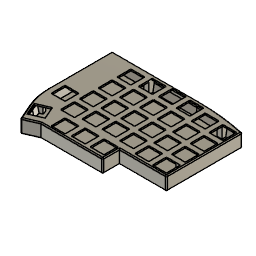
Like Lily58 (Autodesk Fusion 360 design; units mm, degrees)
Autodesk Fusion 360 part; units mm, degrees
(part 1 of 2)
sketch "Plate" plane through (0, 0, 0) normal (0, 0, 1) x (1, 0, 0)
  arc A0 (259.7, -60.0305) -> (260.2, -60.5305) centre (260.2, -60.0305) ccw
  arc A1 (235.6, -61.318) -> (235.1, -60.818) centre (235.1, -61.318) ccw
  line L0 (221.6, -61.318) -> (221.6, -74.318)
  line L1 (222.1, -60.818) -> (235.1, -60.818)
  arc A2 (197, -74.818) -> (197.5, -74.318) centre (197, -74.318) ccw
  line L2 (203.05, -73.675) -> (216.05, -73.675)
  line L3 (159.4, -54.46) -> (159.4, -67.46)
  line L4 (184, -60.818) -> (197, -60.818)
  arc A3 (145.9, -53.96) -> (145.4, -54.46) centre (145.9, -54.46) ccw
  line L5 (184, -74.818) -> (197, -74.818)
  arc A4 (184, -60.818) -> (183.5, -61.318) centre (184, -61.318) ccw
  arc A5 (273.2, -60.5305) -> (273.7, -60.0305) centre (273.2, -60.0305) ccw
  line L6 (235.6, -61.318) -> (235.6, -74.318)
  line L7 (183.5, -61.318) -> (183.5, -74.318)
  arc A6 (183.5, -74.318) -> (184, -74.818) centre (184, -74.318) ccw
  arc A7 (197.5, -61.318) -> (197, -60.818) centre (197, -61.318) ccw
  arc A8 (222.1, -60.818) -> (221.6, -61.318) centre (222.1, -61.318) ccw
  line L8 (273.7, -47.0305) -> (273.7, -60.0305)
  arc A9 (216.55, -60.175) -> (216.05, -59.675) centre (216.05, -60.175) ccw
  line L9 (222.1, -74.818) -> (235.1, -74.818)
  line L10 (197.5, -61.318) -> (197.5, -74.318)
  arc A10 (202.55, -73.175) -> (203.05, -73.675) centre (203.05, -73.175) ccw
  line L11 (259.7, -47.0305) -> (259.7, -60.0305)
  line L12 (260.2, -46.5305) -> (273.2, -46.5305)
  arc A11 (260.2, -46.5305) -> (259.7, -47.0305) centre (260.2, -47.0305) ccw
  line L13 (216.55, -60.175) -> (216.55, -73.175)
  arc A12 (203.05, -59.675) -> (202.55, -60.175) centre (203.05, -60.175) ccw
  line L14 (203.05, -16.525) -> (216.05, -16.525)
  line L15 (260.2, -60.5305) -> (273.2, -60.5305)
  arc A13 (216.05, -16.525) -> (216.55, -16.025) centre (216.05, -16.025) ccw
  line L16 (183.5, -4.168) -> (183.5, -17.168)
  line L17 (197.5, -4.168) -> (197.5, -17.168)
  arc A14 (197.5, -4.168) -> (197, -3.668) centre (197, -4.168) ccw
  arc A15 (197, -17.668) -> (197.5, -17.168) centre (197, -17.168) ccw
  line L18 (216.55, -3.025) -> (216.55, -16.025)
  arc A16 (273.7, -47.0305) -> (273.2, -46.5305) centre (273.2, -47.0305) ccw
  arc A17 (145.4, -67.46) -> (145.9, -67.96) centre (145.9, -67.46) ccw
  arc A18 (159.4, -54.46) -> (158.9, -53.96) centre (158.9, -54.46) ccw
  arc A19 (203.05, -2.525) -> (202.55, -3.025) centre (203.05, -3.025) ccw
  arc A20 (216.55, -3.025) -> (216.05, -2.525) centre (216.05, -3.025) ccw
  arc A21 (158.9, -67.96) -> (159.4, -67.46) centre (158.9, -67.46) ccw
  line L19 (145.9, -67.96) -> (158.9, -67.96)
  line L20 (145.4, -54.46) -> (145.4, -67.46)
  line L21 (145.9, -53.96) -> (158.9, -53.96)
  line L22 (222.1, -3.668) -> (235.1, -3.668)
  line L23 (203.05, -59.675) -> (216.05, -59.675)
  arc A22 (216.05, -73.675) -> (216.55, -73.175) centre (216.05, -73.175) ccw
  line L24 (203.05, -2.525) -> (216.05, -2.525)
  line L25 (184, -3.668) -> (197, -3.668)
  line L26 (202.55, -3.025) -> (202.55, -16.025)
  line L27 (202.55, -60.175) -> (202.55, -73.175)
  line L28 (260.2, -22.4305) -> (273.2, -22.4305)
  line L29 (235.6, -4.168) -> (235.6, -17.168)
  line L30 (164.95, -6.335) -> (177.95, -6.335)
  arc A23 (177.95, -20.335) -> (178.45, -19.835) centre (177.95, -19.835) ccw
  arc A24 (241.15, -7.2875) -> (240.65, -7.7875) centre (241.15, -7.7875) ccw
  line L31 (260.2, -8.4305) -> (273.2, -8.4305)
  line L32 (241.15, -7.2875) -> (254.15, -7.2875)
  line L33 (164.45, -6.835) -> (164.45, -19.835)
  arc A25 (259.7, -21.9305) -> (260.2, -22.4305) centre (260.2, -21.9305) ccw
  arc A26 (222.1, -3.668) -> (221.6, -4.168) centre (222.1, -4.168) ccw
  line L34 (259.7, -8.9305) -> (259.7, -21.9305)
  line L35 (178.45, -6.835) -> (178.45, -19.835)
  line L36 (273.7, -8.9305) -> (273.7, -21.9305)
  arc A27 (254.15, -21.2875) -> (254.65, -20.7875) centre (254.15, -20.7875) ccw
  arc A28 (240.65, -20.7875) -> (241.15, -21.2875) centre (241.15, -20.7875) ccw
  line L37 (221.6, -4.168) -> (221.6, -17.168)
  line L38 (164.95, -20.335) -> (177.95, -20.335)
  arc A29 (254.65, -7.7875) -> (254.15, -7.2875) centre (254.15, -7.7875) ccw
  arc A30 (184, -3.668) -> (183.5, -4.168) centre (184, -4.168) ccw
  line L39 (241.15, -21.2875) -> (254.15, -21.2875)
  arc A31 (164.45, -19.835) -> (164.95, -20.335) centre (164.95, -19.835) ccw
  line L40 (222.1, -17.668) -> (235.1, -17.668)
  arc A32 (178.45, -6.835) -> (177.95, -6.335) centre (177.95, -6.835) ccw
  arc A33 (273.2, -22.4305) -> (273.7, -21.9305) centre (273.2, -21.9305) ccw
  arc A34 (221.6, -17.168) -> (222.1, -17.668) centre (222.1, -17.168) ccw
  arc A35 (235.1, -17.668) -> (235.6, -17.168) centre (235.1, -17.168) ccw
  arc A36 (202.55, -16.025) -> (203.05, -16.525) centre (203.05, -16.025) ccw
  arc A37 (273.7, -8.9305) -> (273.2, -8.4305) centre (273.2, -8.9305) ccw
  arc A38 (164.95, -6.335) -> (164.45, -6.835) centre (164.95, -6.835) ccw
  line L41 (184, -17.668) -> (197, -17.668)
  arc A39 (235.6, -4.168) -> (235.1, -3.668) centre (235.1, -4.168) ccw
  line L42 (240.65, -7.7875) -> (240.65, -20.7875)
  line L43 (254.65, -7.7875) -> (254.65, -20.7875)
  arc A40 (183.5, -17.168) -> (184, -17.668) centre (184, -17.168) ccw
  line L44 (164.45, -25.885) -> (164.45, -38.885)
  arc A41 (164.95, -25.385) -> (164.45, -25.885) centre (164.95, -25.885) ccw
  arc A42 (197, -36.718) -> (197.5, -36.218) centre (197, -36.218) ccw
  arc A43 (178.45, -25.885) -> (177.95, -25.385) centre (177.95, -25.885) ccw
  arc A44 (222.1, -22.718) -> (221.6, -23.218) centre (222.1, -23.218) ccw
  arc A45 (177.95, -39.385) -> (178.45, -38.885) centre (177.95, -38.885) ccw
  arc A46 (260.2, -8.4305) -> (259.7, -8.9305) centre (260.2, -8.9305) ccw
  line L45 (216.55, -22.075) -> (216.55, -35.075)
  line L46 (183.5, -23.218) -> (183.5, -36.218)
  line L47 (203.05, -21.575) -> (216.05, -21.575)
  line L48 (222.1, -36.718) -> (235.1, -36.718)
  arc A47 (197.5, -23.218) -> (197, -22.718) centre (197, -23.218) ccw
  line L49 (164.95, -39.385) -> (177.95, -39.385)
  arc A48 (216.05, -35.575) -> (216.55, -35.075) centre (216.05, -35.075) ccw
  line L50 (178.45, -25.885) -> (178.45, -38.885)
  arc A49 (202.55, -35.075) -> (203.05, -35.575) centre (203.05, -35.075) ccw
  arc A50 (183.5, -36.218) -> (184, -36.718) centre (184, -36.218) ccw
  line L51 (184, -36.718) -> (197, -36.718)
  arc A51 (235.6, -23.218) -> (235.1, -22.718) centre (235.1, -23.218) ccw
  line L52 (222.1, -22.718) -> (235.1, -22.718)
  arc A52 (203.05, -21.575) -> (202.55, -22.075) centre (203.05, -22.075) ccw
  arc A53 (235.1, -36.718) -> (235.6, -36.218) centre (235.1, -36.218) ccw
  line L53 (164.95, -25.385) -> (177.95, -25.385)
  arc A54 (184, -22.718) -> (183.5, -23.218) centre (184, -23.218) ccw
  line L54 (235.6, -23.218) -> (235.6, -36.218)
  line L55 (203.05, -35.575) -> (216.05, -35.575)
  arc A55 (216.55, -22.075) -> (216.05, -21.575) centre (216.05, -22.075) ccw
  line L56 (197.5, -23.218) -> (197.5, -36.218)
  line L57 (184, -22.718) -> (197, -22.718)
  arc A56 (164.45, -38.885) -> (164.95, -39.385) centre (164.95, -38.885) ccw
  line L58 (221.6, -23.218) -> (221.6, -36.218)
  line L59 (216.55, -41.125) -> (216.55, -54.125)
  arc A57 (216.05, -54.625) -> (216.55, -54.125) centre (216.05, -54.125) ccw
  arc A58 (259.7, -40.9805) -> (260.2, -41.4805) centre (260.2, -40.9805) ccw
  line L60 (241.15, -40.3375) -> (254.15, -40.3375)
  line L61 (203.05, -54.625) -> (216.05, -54.625)
  line L62 (202.55, -22.075) -> (202.55, -35.075)
  arc A59 (273.7, -27.9805) -> (273.2, -27.4805) centre (273.2, -27.9805) ccw
  line L63 (184, -55.768) -> (197, -55.768)
  line L64 (260.2, -41.4805) -> (273.2, -41.4805)
  line L65 (259.7, -27.9805) -> (259.7, -40.9805)
  arc A60 (202.55, -54.125) -> (203.05, -54.625) centre (203.05, -54.125) ccw
  arc A61 (203.05, -40.625) -> (202.55, -41.125) centre (203.05, -41.125) ccw
  arc A62 (254.15, -40.3375) -> (254.65, -39.8375) centre (254.15, -39.8375) ccw
  line L66 (240.65, -26.8375) -> (240.65, -39.8375)
  arc A63 (221.6, -36.218) -> (222.1, -36.718) centre (222.1, -36.218) ccw
  arc A64 (240.65, -39.8375) -> (241.15, -40.3375) centre (241.15, -39.8375) ccw
  line L67 (203.05, -40.625) -> (216.05, -40.625)
  arc A65 (273.2, -41.4805) -> (273.7, -40.9805) centre (273.2, -40.9805) ccw
  line L68 (241.15, -26.3375) -> (254.15, -26.3375)
  arc A66 (254.65, -26.8375) -> (254.15, -26.3375) centre (254.15, -26.8375) ccw
  line L69 (184, -41.768) -> (197, -41.768)
  line L70 (183.5, -42.268) -> (183.5, -55.268)
  line L71 (197.5, -42.268) -> (197.5, -55.268)
  arc A67 (216.55, -41.125) -> (216.05, -40.625) centre (216.05, -41.125) ccw
  arc A68 (184, -41.768) -> (183.5, -42.268) centre (184, -42.268) ccw
  line L72 (273.7, -27.9805) -> (273.7, -40.9805)
  arc A69 (260.2, -27.4805) -> (259.7, -27.9805) centre (260.2, -27.9805) ccw
  arc A70 (241.15, -26.3375) -> (240.65, -26.8375) centre (241.15, -26.8375) ccw
  line L73 (202.55, -41.125) -> (202.55, -54.125)
  arc A71 (177.95, -58.435) -> (178.45, -57.935) centre (177.95, -57.935) ccw
  arc A72 (221.6, -55.268) -> (222.1, -55.768) centre (222.1, -55.268) ccw
  line L74 (164.45, -44.935) -> (164.45, -57.935)
  line L75 (241.15, -45.3875) -> (254.15, -45.3875)
  arc A73 (235.1, -55.768) -> (235.6, -55.268) centre (235.1, -55.268) ccw
  line L76 (241.15, -59.3875) -> (254.15, -59.3875)
  line L77 (254.65, -45.8875) -> (254.65, -58.8875)
  line L78 (164.95, -44.435) -> (177.95, -44.435)
  arc A74 (240.65, -58.8875) -> (241.15, -59.3875) centre (241.15, -58.8875) ccw
  line L79 (178.45, -44.935) -> (178.45, -57.935)
  line L80 (222.1, -41.768) -> (235.1, -41.768)
  line L81 (254.65, -26.8375) -> (254.65, -39.8375)
  line L82 (240.65, -45.8875) -> (240.65, -58.8875)
  arc A75 (178.45, -44.935) -> (177.95, -44.435) centre (177.95, -44.935) ccw
  line L83 (222.1, -55.768) -> (235.1, -55.768)
  line L84 (164.95, -58.435) -> (177.95, -58.435)
  arc A76 (254.65, -45.8875) -> (254.15, -45.3875) centre (254.15, -45.8875) ccw
  line L85 (235.6, -42.268) -> (235.6, -55.268)
  arc A77 (183.5, -55.268) -> (184, -55.768) centre (184, -55.268) ccw
  arc A78 (241.15, -45.3875) -> (240.65, -45.8875) centre (241.15, -45.8875) ccw
  arc A79 (235.6, -42.268) -> (235.1, -41.768) centre (235.1, -42.268) ccw
  arc A80 (222.1, -41.768) -> (221.6, -42.268) centre (222.1, -42.268) ccw
  arc A81 (164.45, -57.935) -> (164.95, -58.435) centre (164.95, -57.935) ccw
  line L86 (221.6, -42.268) -> (221.6, -55.268)
  line L87 (260.2, -27.4805) -> (273.2, -27.4805)
  arc A82 (254.15, -59.3875) -> (254.65, -58.8875) centre (254.15, -58.8875) ccw
  arc A83 (177.95, -77.485) -> (178.45, -76.985) centre (177.95, -76.985) ccw
  arc A84 (197.5, -42.268) -> (197, -41.768) centre (197, -42.268) ccw
  line L88 (241.15, -64.4375) -> (254.15, -64.4375)
  arc A85 (273.7, -66.0805) -> (273.2, -65.5805) centre (273.2, -66.0805) ccw
  line L89 (164.95, -63.485) -> (177.95, -63.485)
  arc A86 (197, -55.768) -> (197.5, -55.268) centre (197, -55.268) ccw
  arc A87 (178.45, -63.985) -> (177.95, -63.485) centre (177.95, -63.985) ccw
  line L90 (260.2, -65.5805) -> (273.2, -65.5805)
  arc A88 (164.95, -44.435) -> (164.45, -44.935) centre (164.95, -44.935) ccw
  arc A89 (260.2, -65.5805) -> (259.7, -66.0805) centre (260.2, -66.0805) ccw
  line L91 (241.15, -78.4375) -> (254.15, -78.4375)
  arc A90 (259.7, -79.0805) -> (260.2, -79.5805) centre (260.2, -79.0805) ccw
  line L92 (254.65, -64.9375) -> (254.65, -77.9375)
  line L93 (164.45, -63.985) -> (164.45, -76.985)
  arc A91 (221.6, -74.318) -> (222.1, -74.818) centre (222.1, -74.318) ccw
  arc A92 (235.1, -74.818) -> (235.6, -74.318) centre (235.1, -74.318) ccw
  line L94 (164.95, -77.485) -> (177.95, -77.485)
  line L95 (178.45, -63.985) -> (178.45, -76.985)
  line L96 (259.7, -66.0805) -> (259.7, -79.0805)
  arc A93 (241.15, -64.4375) -> (240.65, -64.9375) centre (241.15, -64.9375) ccw
  line L97 (273.7, -66.0805) -> (273.7, -79.0805)
  arc A94 (164.95, -63.485) -> (164.45, -63.985) centre (164.95, -63.985) ccw
  arc A95 (254.65, -64.9375) -> (254.15, -64.4375) centre (254.15, -64.9375) ccw
  arc A96 (273.2, -79.5805) -> (273.7, -79.0805) centre (273.2, -79.0805) ccw
  arc A97 (254.15, -78.4375) -> (254.65, -77.9375) centre (254.15, -77.9375) ccw
  line L98 (240.65, -64.9375) -> (240.65, -77.9375)
  arc A98 (164.45, -76.985) -> (164.95, -77.485) centre (164.95, -76.985) ccw
  line L99 (260.2, -79.5805) -> (273.2, -79.5805)
  arc A99 (240.65, -77.9375) -> (241.15, -78.4375) centre (241.15, -77.9375) ccw
  line L100 (193.525, -81.2015) -> (206.525, -81.2015)
  line L101 (187.975, -83.035) -> (187.975, -96.035)
  arc A100 (193.025, -94.7015) -> (193.525, -95.2015) centre (193.525, -94.7015) ccw
  arc A101 (187.975, -83.035) -> (187.475, -82.535) centre (187.475, -83.035) ccw
  arc A102 (206.525, -95.2015) -> (207.025, -94.7015) centre (206.525, -94.7015) ccw
  line L102 (174.475, -82.535) -> (187.475, -82.535)
  arc A103 (225.575, -95.2015) -> (226.075, -94.7015) centre (225.575, -94.7015) ccw
  line L103 (212.575, -81.2015) -> (225.575, -81.2015)
  arc A104 (212.075, -94.7015) -> (212.575, -95.2015) centre (212.575, -94.7015) ccw
  line L104 (193.025, -81.7015) -> (193.025, -94.7015)
  arc A105 (174.475, -82.535) -> (173.975, -83.035) centre (174.475, -83.035) ccw
  line L105 (173.975, -83.035) -> (173.975, -96.035)
  arc A106 (207.025, -81.7015) -> (206.525, -81.2015) centre (206.525, -81.7015) ccw
  line L106 (207.025, -81.7015) -> (207.025, -94.7015)
  arc A107 (226.075, -81.7015) -> (225.575, -81.2015) centre (225.575, -81.7015) ccw
  line L107 (212.075, -81.7015) -> (212.075, -94.7015)
  line L108 (212.575, -95.2015) -> (225.575, -95.2015)
  arc A108 (187.475, -96.535) -> (187.975, -96.035) centre (187.475, -96.035) ccw
  arc A109 (173.975, -96.035) -> (174.475, -96.535) centre (174.475, -96.035) ccw
  arc A110 (193.525, -81.2015) -> (193.025, -81.7015) centre (193.525, -81.7015) ccw
  line L109 (174.475, -96.535) -> (187.475, -96.535)
  line L110 (226.075, -81.7015) -> (226.075, -94.7015)
  arc A111 (212.575, -81.2015) -> (212.075, -81.7015) centre (212.575, -81.7015) ccw
  line L111 (193.525, -95.2015) -> (206.525, -95.2015)
  line L112 (226.8375, -0.025) -> (139.1942, -0.025)
  line L113 (276.2, -82.0805) -> (276.2, -5.454)
  arc A112 (276.2, -5.454) -> (226.8375, -0.025) centre (226.8375, -227.1492) ccw
  line L114 (276.2, -82.0805) -> (228.575, -82.0805)
  line L115 (165.9817, -99.035) -> (228.575, -99.035)
  line L116 (228.575, -99.035) -> (228.575, -82.0805)
  line L117 (145.666, -85.4803) -> (158.518, -79.9282)
  line L118 (158.518, -79.9282) -> (164.0701, -92.7802)
  line L119 (164.0701, -92.7802) -> (151.218, -98.3323)
  line L120 (151.218, -98.3323) -> (145.666, -85.4803)
  line L121 (139.1942, -0.025) -> (139.1942, -64.9159)
  line L122 (165.9817, -99.035) -> (151.5008, -105.2907)
  line L123 (151.5008, -105.2907) -> (143.9083, -87.7156)
  arc A113 (139.1942, -64.9159) -> (143.9083, -87.7156) centre (196.6857, -64.9159) ccw
  dimension "d8" = 2.5
  dimension "d9" = 2.5
  dimension "d11" = 2.5
  dimension "d12" = 2.5
  dimension "d13" = 2.5
  dimension "d24" = 2.5
  dimension "d29" = 6.5
  constraint tangent L112 A112
  constraint parallel L24 L112
  constraint perpendicular L113 L114
  constraint horizontal L115
  constraint perpendicular L114 L116
  constraint perpendicular L112 L121
  constraint tangent L123 A113
  constraint tangent L121 A113
  constraint parallel L120 L123
  constraint parallel L119 L122
  measures "d8" distance of L24 L112
  measures "d9" distance of L72 L113
  measures "d11" distance of L109 L115
  measures "d12" distance of L110 L116
  measures "d13" distance of L99 L114
  measures "d24" distance of L120 L123
  measures "d29" distance of L119 L122
extrude "Extrude1" add sketch "Plate" against normal blind 3.5 thin wall 1.7 inside contours A0 A5 L8 L11 L12 A11 L15 A16 | A1 L0 L1 L6 A8 L9 A91 A92 | A2 L4 L5 A4 L7 A6 A7 L10 | L2 A9 A10 L13 A12 L23 A22 L27 | L3 A3 A17 A18 A21 L19 L20 L21 | L14 A13 L18 A19 A20 L24 L26 A36 | L16 L17 A14 A15 L25 A30 L41 A40 | L22 L29 A26 L37 L40 A34 A35 A39 | L28 L31 A25 L34 L36 A33 A37 A46 | L30 A23 L33 L35 L38 A31 A32 A38 | A24 L32 A27 A28 A29 L39 L42 L43 | L44 A41 A43 A45 L49 L50 L53 A56 | A42 L46 A47 A50 L51 A54 L56 L57 | A44 L48 A51 L52 A53 L54 L58 A63 | L45 L47 A48 A49 A52 L55 A55 L62 | L59 A57 L61 A60 A61 L67 A67 L73 | A58 A59 L64 L65 A65 L72 A69 L87 | L60 A62 L66 A64 L68 A66 A70 L81 | L63 L69 L70 L71 A68 A77 A84 A86 | A71 L74 L78 L79 A75 L84 A81 A88 | A72 A73 L80 L83 L85 A79 A80 L86 | L75 L76 L77 A74 L82 A76 A78 A82 | A83 L89 A87 L93 L94 L95 A94 A98 | L88 L91 L92 A93 A95 A97 L98 A99 | A85 L90 A89 A90 L96 L97 A96 L99 | L100 A100 A102 L104 A106 L106 A110 L111 | L101 A101 L102 A105 L105 A108 A109 L109 | A103 L103 A104 A107 L107 L108 L110 A111 | L112 L113 A112 L114 L115 L116 L121 L122 L123 A113 | L117 L118 L119 L120 makes body 1
extrude "Extrude2" add sketch "Plate" along normal blind 1.5 bodies 1
extrude "Extrude3" add 1 faces at (168.9753, -0.5917, -3.5) along direction (0, 0, -1) blind 7.5 draft 10 on bodies 1 bodies 1
sketch "Sketch5" plane through (0, 0, 1.5) normal (0, 0, 1) x (-1, 0, 0)
  line L0 (-164.0701, 92.7802) -> (-151.218, 98.3323)
  line L1 (-151.218, 98.3323) -> (-145.666, 85.4803)
  line L2 (-145.666, 85.4803) -> (-158.518, 79.9282)
  line L3 (-158.518, 79.9282) -> (-164.0701, 92.7802)
  arc A0 (-260.2, 65.5805) -> (-259.7, 66.0805) centre (-260.2, 66.0805) ccw
  line L4 (-260.2, 65.5805) -> (-273.2, 65.5805)
  arc A1 (-273.7, 66.0805) -> (-273.2, 65.5805) centre (-273.2, 66.0805) ccw
  line L5 (-273.7, 66.0805) -> (-273.7, 79.0805)
  arc A2 (-273.2, 79.5805) -> (-273.7, 79.0805) centre (-273.2, 79.0805) ccw
  line L6 (-273.2, 79.5805) -> (-260.2, 79.5805)
  arc A3 (-259.7, 79.0805) -> (-260.2, 79.5805) centre (-260.2, 79.0805) ccw
  line L7 (-259.7, 79.0805) -> (-259.7, 66.0805)
  arc A4 (-174.475, 82.535) -> (-173.975, 83.035) centre (-174.475, 83.035) ccw
  line L8 (-174.475, 82.535) -> (-187.475, 82.535)
  arc A5 (-187.975, 83.035) -> (-187.475, 82.535) centre (-187.475, 83.035) ccw
  line L9 (-187.975, 83.035) -> (-187.975, 96.035)
  arc A6 (-187.475, 96.535) -> (-187.975, 96.035) centre (-187.475, 96.035) ccw
  line L10 (-187.475, 96.535) -> (-174.475, 96.535)
  arc A7 (-173.975, 96.035) -> (-174.475, 96.535) centre (-174.475, 96.035) ccw
  line L11 (-173.975, 96.035) -> (-173.975, 83.035)
  arc A8 (-203.05, 59.675) -> (-202.55, 60.175) centre (-203.05, 60.175) ccw
  line L12 (-203.05, 59.675) -> (-216.05, 59.675)
  arc A9 (-216.55, 60.175) -> (-216.05, 59.675) centre (-216.05, 60.175) ccw
  line L13 (-216.55, 60.175) -> (-216.55, 73.175)
  arc A10 (-216.05, 73.675) -> (-216.55, 73.175) centre (-216.05, 73.175) ccw
  line L14 (-216.05, 73.675) -> (-203.05, 73.675)
  arc A11 (-202.55, 73.175) -> (-203.05, 73.675) centre (-203.05, 73.175) ccw
  line L15 (-202.55, 73.175) -> (-202.55, 60.175)
  arc A12 (-260.2, 46.5305) -> (-259.7, 47.0305) centre (-260.2, 47.0305) ccw
  line L16 (-260.2, 46.5305) -> (-273.2, 46.5305)
  arc A13 (-273.7, 47.0305) -> (-273.2, 46.5305) centre (-273.2, 47.0305) ccw
  line L17 (-273.7, 47.0305) -> (-273.7, 60.0305)
  arc A14 (-273.2, 60.5305) -> (-273.7, 60.0305) centre (-273.2, 60.0305) ccw
  line L18 (-273.2, 60.5305) -> (-260.2, 60.5305)
  arc A15 (-259.7, 60.0305) -> (-260.2, 60.5305) centre (-260.2, 60.0305) ccw
  line L19 (-259.7, 60.0305) -> (-259.7, 47.0305)
  arc A16 (-241.15, 64.4375) -> (-240.65, 64.9375) centre (-241.15, 64.9375) ccw
  line L20 (-241.15, 64.4375) -> (-254.15, 64.4375)
  arc A17 (-254.65, 64.9375) -> (-254.15, 64.4375) centre (-254.15, 64.9375) ccw
  line L21 (-254.65, 64.9375) -> (-254.65, 77.9375)
  arc A18 (-254.15, 78.4375) -> (-254.65, 77.9375) centre (-254.15, 77.9375) ccw
  line L22 (-254.15, 78.4375) -> (-241.15, 78.4375)
  arc A19 (-240.65, 77.9375) -> (-241.15, 78.4375) centre (-241.15, 77.9375) ccw
  line L23 (-240.65, 77.9375) -> (-240.65, 64.9375)
  arc A20 (-164.95, 63.485) -> (-164.45, 63.985) centre (-164.95, 63.985) ccw
  line L24 (-164.95, 63.485) -> (-177.95, 63.485)
  arc A21 (-178.45, 63.985) -> (-177.95, 63.485) centre (-177.95, 63.985) ccw
  line L25 (-178.45, 63.985) -> (-178.45, 76.985)
  arc A22 (-177.95, 77.485) -> (-178.45, 76.985) centre (-177.95, 76.985) ccw
  line L26 (-177.95, 77.485) -> (-164.95, 77.485)
  arc A23 (-164.45, 76.985) -> (-164.95, 77.485) centre (-164.95, 76.985) ccw
  line L27 (-164.45, 76.985) -> (-164.45, 63.985)
  arc A24 (-222.1, 60.818) -> (-221.6, 61.318) centre (-222.1, 61.318) ccw
  line L28 (-222.1, 60.818) -> (-235.1, 60.818)
  arc A25 (-235.6, 61.318) -> (-235.1, 60.818) centre (-235.1, 61.318) ccw
  line L29 (-235.6, 61.318) -> (-235.6, 74.318)
  arc A26 (-235.1, 74.818) -> (-235.6, 74.318) centre (-235.1, 74.318) ccw
  line L30 (-235.1, 74.818) -> (-222.1, 74.818)
  arc A27 (-221.6, 74.318) -> (-222.1, 74.818) centre (-222.1, 74.318) ccw
  line L31 (-221.6, 74.318) -> (-221.6, 61.318)
  arc A28 (-226.075, 81.7015) -> (-225.575, 81.2015) centre (-225.575, 81.7015) ccw
  line L32 (-226.075, 81.7015) -> (-226.075, 94.7015)
  arc A29 (-225.575, 95.2015) -> (-226.075, 94.7015) centre (-225.575, 94.7015) ccw
  line L33 (-225.575, 95.2015) -> (-212.575, 95.2015)
  arc A30 (-212.075, 94.7015) -> (-212.575, 95.2015) centre (-212.575, 94.7015) ccw
  line L34 (-212.075, 94.7015) -> (-212.075, 81.7015)
  arc A31 (-212.575, 81.2015) -> (-212.075, 81.7015) centre (-212.575, 81.7015) ccw
  line L35 (-212.575, 81.2015) -> (-225.575, 81.2015)
  arc A32 (-193.525, 81.2015) -> (-193.025, 81.7015) centre (-193.525, 81.7015) ccw
  line L36 (-193.525, 81.2015) -> (-206.525, 81.2015)
  arc A33 (-207.025, 81.7015) -> (-206.525, 81.2015) centre (-206.525, 81.7015) ccw
  line L37 (-207.025, 81.7015) -> (-207.025, 94.7015)
  arc A34 (-206.525, 95.2015) -> (-207.025, 94.7015) centre (-206.525, 94.7015) ccw
  line L38 (-206.525, 95.2015) -> (-193.525, 95.2015)
  arc A35 (-193.025, 94.7015) -> (-193.525, 95.2015) centre (-193.525, 94.7015) ccw
  line L39 (-193.025, 94.7015) -> (-193.025, 81.7015)
  arc A36 (-178.45, 44.935) -> (-177.95, 44.435) centre (-177.95, 44.935) ccw
  line L40 (-178.45, 44.935) -> (-178.45, 57.935)
  arc A37 (-177.95, 58.435) -> (-178.45, 57.935) centre (-177.95, 57.935) ccw
  line L41 (-177.95, 58.435) -> (-164.95, 58.435)
  arc A38 (-164.45, 57.935) -> (-164.95, 58.435) centre (-164.95, 57.935) ccw
  line L42 (-164.45, 57.935) -> (-164.45, 44.935)
  arc A39 (-164.95, 44.435) -> (-164.45, 44.935) centre (-164.95, 44.935) ccw
  line L43 (-164.95, 44.435) -> (-177.95, 44.435)
  arc A40 (-241.15, 45.3875) -> (-240.65, 45.8875) centre (-241.15, 45.8875) ccw
  line L44 (-241.15, 45.3875) -> (-254.15, 45.3875)
  arc A41 (-254.65, 45.8875) -> (-254.15, 45.3875) centre (-254.15, 45.8875) ccw
  line L45 (-254.65, 45.8875) -> (-254.65, 58.8875)
  arc A42 (-254.15, 59.3875) -> (-254.65, 58.8875) centre (-254.15, 58.8875) ccw
  line L46 (-254.15, 59.3875) -> (-241.15, 59.3875)
  arc A43 (-240.65, 58.8875) -> (-241.15, 59.3875) centre (-241.15, 58.8875) ccw
  line L47 (-240.65, 58.8875) -> (-240.65, 45.8875)
  arc A44 (-184, 41.768) -> (-183.5, 42.268) centre (-184, 42.268) ccw
  line L48 (-184, 41.768) -> (-197, 41.768)
  arc A45 (-197.5, 42.268) -> (-197, 41.768) centre (-197, 42.268) ccw
  line L49 (-197.5, 42.268) -> (-197.5, 55.268)
  arc A46 (-197, 55.768) -> (-197.5, 55.268) centre (-197, 55.268) ccw
  line L50 (-197, 55.768) -> (-184, 55.768)
  arc A47 (-183.5, 55.268) -> (-184, 55.768) centre (-184, 55.268) ccw
  line L51 (-183.5, 55.268) -> (-183.5, 42.268)
  line L52 (-259.7, 40.9805) -> (-259.7, 27.9805)
  arc A48 (-260.2, 27.4805) -> (-259.7, 27.9805) centre (-260.2, 27.9805) ccw
  line L53 (-260.2, 27.4805) -> (-273.2, 27.4805)
  arc A49 (-273.7, 27.9805) -> (-273.2, 27.4805) centre (-273.2, 27.9805) ccw
  line L54 (-273.7, 27.9805) -> (-273.7, 40.9805)
  arc A50 (-273.2, 41.4805) -> (-273.7, 40.9805) centre (-273.2, 40.9805) ccw
  line L55 (-273.2, 41.4805) -> (-260.2, 41.4805)
  arc A51 (-259.7, 40.9805) -> (-260.2, 41.4805) centre (-260.2, 40.9805) ccw
  arc A52 (-222.1, 41.768) -> (-221.6, 42.268) centre (-222.1, 42.268) ccw
  line L56 (-222.1, 41.768) -> (-235.1, 41.768)
  arc A53 (-235.6, 42.268) -> (-235.1, 41.768) centre (-235.1, 42.268) ccw
  line L57 (-235.6, 42.268) -> (-235.6, 55.268)
  arc A54 (-235.1, 55.768) -> (-235.6, 55.268) centre (-235.1, 55.268) ccw
  line L58 (-235.1, 55.768) -> (-222.1, 55.768)
  arc A55 (-221.6, 55.268) -> (-222.1, 55.768) centre (-222.1, 55.268) ccw
  line L59 (-221.6, 55.268) -> (-221.6, 42.268)
  arc A56 (-203.05, 40.625) -> (-202.55, 41.125) centre (-203.05, 41.125) ccw
  line L60 (-203.05, 40.625) -> (-216.05, 40.625)
  arc A57 (-216.55, 41.125) -> (-216.05, 40.625) centre (-216.05, 41.125) ccw
  line L61 (-216.55, 41.125) -> (-216.55, 54.125)
  arc A58 (-216.05, 54.625) -> (-216.55, 54.125) centre (-216.05, 54.125) ccw
  line L62 (-216.05, 54.625) -> (-203.05, 54.625)
  arc A59 (-202.55, 54.125) -> (-203.05, 54.625) centre (-203.05, 54.125) ccw
  line L63 (-202.55, 54.125) -> (-202.55, 41.125)
  arc A60 (-222.1, 22.718) -> (-221.6, 23.218) centre (-222.1, 23.218) ccw
  line L64 (-222.1, 22.718) -> (-235.1, 22.718)
  arc A61 (-235.6, 23.218) -> (-235.1, 22.718) centre (-235.1, 23.218) ccw
  line L65 (-235.6, 23.218) -> (-235.6, 36.218)
  arc A62 (-235.1, 36.718) -> (-235.6, 36.218) centre (-235.1, 36.218) ccw
  line L66 (-235.1, 36.718) -> (-222.1, 36.718)
  arc A63 (-221.6, 36.218) -> (-222.1, 36.718) centre (-222.1, 36.218) ccw
  line L67 (-221.6, 36.218) -> (-221.6, 23.218)
  arc A64 (-241.15, 26.3375) -> (-240.65, 26.8375) centre (-241.15, 26.8375) ccw
  line L68 (-241.15, 26.3375) -> (-254.15, 26.3375)
  arc A65 (-254.65, 26.8375) -> (-254.15, 26.3375) centre (-254.15, 26.8375) ccw
  line L69 (-254.65, 26.8375) -> (-254.65, 39.8375)
  arc A66 (-254.15, 40.3375) -> (-254.65, 39.8375) centre (-254.15, 39.8375) ccw
  line L70 (-254.15, 40.3375) -> (-241.15, 40.3375)
  arc A67 (-240.65, 39.8375) -> (-241.15, 40.3375) centre (-241.15, 39.8375) ccw
  line L71 (-240.65, 39.8375) -> (-240.65, 26.8375)
  arc A68 (-203.05, 21.575) -> (-202.55, 22.075) centre (-203.05, 22.075) ccw
  line L72 (-203.05, 21.575) -> (-216.05, 21.575)
  arc A69 (-216.55, 22.075) -> (-216.05, 21.575) centre (-216.05, 22.075) ccw
  line L73 (-216.55, 22.075) -> (-216.55, 35.075)
  arc A70 (-216.05, 35.575) -> (-216.55, 35.075) centre (-216.05, 35.075) ccw
  line L74 (-216.05, 35.575) -> (-203.05, 35.575)
  arc A71 (-202.55, 35.075) -> (-203.05, 35.575) centre (-203.05, 35.075) ccw
  line L75 (-202.55, 35.075) -> (-202.55, 22.075)
  arc A72 (-164.95, 25.385) -> (-164.45, 25.885) centre (-164.95, 25.885) ccw
  line L76 (-164.95, 25.385) -> (-177.95, 25.385)
  arc A73 (-178.45, 25.885) -> (-177.95, 25.385) centre (-177.95, 25.885) ccw
  line L77 (-178.45, 25.885) -> (-178.45, 38.885)
  arc A74 (-177.95, 39.385) -> (-178.45, 38.885) centre (-177.95, 38.885) ccw
  line L78 (-177.95, 39.385) -> (-164.95, 39.385)
  arc A75 (-164.45, 38.885) -> (-164.95, 39.385) centre (-164.95, 38.885) ccw
  line L79 (-164.45, 38.885) -> (-164.45, 25.885)
  line L80 (-183.5, 36.218) -> (-183.5, 23.218)
  arc A76 (-184, 22.718) -> (-183.5, 23.218) centre (-184, 23.218) ccw
  line L81 (-184, 22.718) -> (-197, 22.718)
  arc A77 (-197.5, 23.218) -> (-197, 22.718) centre (-197, 23.218) ccw
  line L82 (-197.5, 23.218) -> (-197.5, 36.218)
  arc A78 (-197, 36.718) -> (-197.5, 36.218) centre (-197, 36.218) ccw
  line L83 (-197, 36.718) -> (-184, 36.718)
  arc A79 (-183.5, 36.218) -> (-184, 36.718) centre (-184, 36.218) ccw
  arc A80 (-184, 60.818) -> (-183.5, 61.318) centre (-184, 61.318) ccw
  line L84 (-184, 60.818) -> (-197, 60.818)
  arc A81 (-197.5, 61.318) -> (-197, 60.818) centre (-197, 61.318) ccw
  line L85 (-197.5, 61.318) -> (-197.5, 74.318)
  arc A82 (-197, 74.818) -> (-197.5, 74.318) centre (-197, 74.318) ccw
  line L86 (-197, 74.818) -> (-184, 74.818)
  arc A83 (-183.5, 74.318) -> (-184, 74.818) centre (-184, 74.318) ccw
  line L87 (-183.5, 74.318) -> (-183.5, 61.318)
  line L88 (-145.4, 67.46) -> (-145.4, 54.46)
  arc A84 (-145.9, 53.96) -> (-145.4, 54.46) centre (-145.9, 54.46) ccw
  line L89 (-145.9, 53.96) -> (-158.9, 53.96)
  arc A85 (-159.4, 54.46) -> (-158.9, 53.96) centre (-158.9, 54.46) ccw
  line L90 (-159.4, 54.46) -> (-159.4, 67.46)
  arc A86 (-158.9, 67.96) -> (-159.4, 67.46) centre (-158.9, 67.46) ccw
  line L91 (-158.9, 67.96) -> (-145.9, 67.96)
  arc A87 (-145.4, 67.46) -> (-145.9, 67.96) centre (-145.9, 67.46) ccw
  arc A88 (-241.15, 7.2875) -> (-240.65, 7.7875) centre (-241.15, 7.7875) ccw
  line L92 (-241.15, 7.2875) -> (-254.15, 7.2875)
  arc A89 (-254.65, 7.7875) -> (-254.15, 7.2875) centre (-254.15, 7.7875) ccw
  line L93 (-254.65, 7.7875) -> (-254.65, 20.7875)
  arc A90 (-254.15, 21.2875) -> (-254.65, 20.7875) centre (-254.15, 20.7875) ccw
  line L94 (-254.15, 21.2875) -> (-241.15, 21.2875)
  arc A91 (-240.65, 20.7875) -> (-241.15, 21.2875) centre (-241.15, 20.7875) ccw
  line L95 (-240.65, 20.7875) -> (-240.65, 7.7875)
  arc A92 (-222.1, 3.668) -> (-221.6, 4.168) centre (-222.1, 4.168) ccw
  line L96 (-222.1, 3.668) -> (-235.1, 3.668)
  arc A93 (-235.6, 4.168) -> (-235.1, 3.668) centre (-235.1, 4.168) ccw
  line L97 (-235.6, 4.168) -> (-235.6, 17.168)
  arc A94 (-235.1, 17.668) -> (-235.6, 17.168) centre (-235.1, 17.168) ccw
  line L98 (-235.1, 17.668) -> (-222.1, 17.668)
  arc A95 (-221.6, 17.168) -> (-222.1, 17.668) centre (-222.1, 17.168) ccw
  line L99 (-221.6, 17.168) -> (-221.6, 4.168)
  arc A96 (-178.45, 6.835) -> (-177.95, 6.335) centre (-177.95, 6.835) ccw
  line L100 (-178.45, 6.835) -> (-178.45, 19.835)
  arc A97 (-177.95, 20.335) -> (-178.45, 19.835) centre (-177.95, 19.835) ccw
  line L101 (-177.95, 20.335) -> (-164.95, 20.335)
  arc A98 (-164.45, 19.835) -> (-164.95, 20.335) centre (-164.95, 19.835) ccw
  line L102 (-164.45, 19.835) -> (-164.45, 6.835)
  arc A99 (-164.95, 6.335) -> (-164.45, 6.835) centre (-164.95, 6.835) ccw
  line L103 (-164.95, 6.335) -> (-177.95, 6.335)
  arc A100 (-203.05, 2.525) -> (-202.55, 3.025) centre (-203.05, 3.025) ccw
  line L104 (-203.05, 2.525) -> (-216.05, 2.525)
  arc A101 (-216.55, 3.025) -> (-216.05, 2.525) centre (-216.05, 3.025) ccw
  line L105 (-216.55, 3.025) -> (-216.55, 16.025)
  arc A102 (-216.05, 16.525) -> (-216.55, 16.025) centre (-216.05, 16.025) ccw
  line L106 (-216.05, 16.525) -> (-203.05, 16.525)
  arc A103 (-202.55, 16.025) -> (-203.05, 16.525) centre (-203.05, 16.025) ccw
  line L107 (-202.55, 16.025) -> (-202.55, 3.025)
  arc A104 (-273.7, 8.9305) -> (-273.2, 8.4305) centre (-273.2, 8.9305) ccw
  line L108 (-273.7, 8.9305) -> (-273.7, 21.9305)
  arc A105 (-273.2, 22.4305) -> (-273.7, 21.9305) centre (-273.2, 21.9305) ccw
  line L109 (-273.2, 22.4305) -> (-260.2, 22.4305)
  arc A106 (-259.7, 21.9305) -> (-260.2, 22.4305) centre (-260.2, 21.9305) ccw
  line L110 (-259.7, 21.9305) -> (-259.7, 8.9305)
  arc A107 (-260.2, 8.4305) -> (-259.7, 8.9305) centre (-260.2, 8.9305) ccw
  line L111 (-260.2, 8.4305) -> (-273.2, 8.4305)
  arc A108 (-184, 3.668) -> (-183.5, 4.168) centre (-184, 4.168) ccw
  line L112 (-184, 3.668) -> (-197, 3.668)
  arc A109 (-197.5, 4.168) -> (-197, 3.668) centre (-197, 4.168) ccw
  line L113 (-197.5, 4.168) -> (-197.5, 17.168)
  arc A110 (-197, 17.668) -> (-197.5, 17.168) centre (-197, 17.168) ccw
  line L114 (-197, 17.668) -> (-184, 17.668)
  arc A111 (-183.5, 17.168) -> (-184, 17.668) centre (-184, 17.168) ccw
  line L115 (-183.5, 17.168) -> (-183.5, 4.168)
  line L116 (-276.2, 82.0805) -> (-276.2, 5.454)
  arc A112 (-276.2, 5.454) -> (-226.8375, 0.025) centre (-226.8375, 227.1492) ccw
  line L117 (-226.8375, 0.025) -> (-139.1942, 0.025)
  line L118 (-139.1942, 0.025) -> (-139.1942, 64.9159)
  arc A113 (-139.1942, 64.9159) -> (-143.9083, 87.7156) centre (-196.6857, 64.9159) ccw
  line L119 (-143.9083, 87.7156) -> (-151.5008, 105.2907)
  line L120 (-151.5008, 105.2907) -> (-165.9817, 99.035)
  line L121 (-165.9817, 99.035) -> (-228.575, 99.035)
  line L122 (-228.575, 99.035) -> (-228.575, 82.0805)
  line L123 (-228.575, 82.0805) -> (-276.2, 82.0805)
  line L124 (-126.932, -12.1644) -> (-288.3358, -12.1644)
  line L125 (-288.3358, -12.1644) -> (-288.3358, 119.2108)
  line L126 (-288.3358, 119.2108) -> (-126.932, 119.2108)
  line L127 (-126.932, 119.2108) -> (-126.932, -12.1644)
  constraint horizontal L124
  constraint vertical L125
  constraint horizontal L126
  constraint vertical L127
extrude "Extrude4" cut sketch "Sketch5" against normal blind 55 contours L124 L125 L126 L127 bodies 1
sketch "Sketch6" plane through (0, 0, 0) normal (0, 0, -1) x (1, 0, 0)
  arc A0 (183.5, 4.168) -> (184, 3.668) centre (184, 4.168) ccw
  line L0 (183.5, 4.168) -> (183.5, 17.168)
  arc A1 (184, 17.668) -> (183.5, 17.168) centre (184, 17.168) ccw
  line L1 (184, 17.668) -> (197, 17.668)
  arc A2 (197.5, 17.168) -> (197, 17.668) centre (197, 17.168) ccw
  line L2 (197.5, 17.168) -> (197.5, 4.168)
  arc A3 (197, 3.668) -> (197.5, 4.168) centre (197, 4.168) ccw
  line L3 (197, 3.668) -> (184, 3.668)
  arc A4 (273.2, 8.4305) -> (273.7, 8.9305) centre (273.2, 8.9305) ccw
  line L4 (273.2, 8.4305) -> (260.2, 8.4305)
  arc A5 (259.7, 8.9305) -> (260.2, 8.4305) centre (260.2, 8.9305) ccw
  line L5 (259.7, 8.9305) -> (259.7, 21.9305)
  arc A6 (260.2, 22.4305) -> (259.7, 21.9305) centre (260.2, 21.9305) ccw
  line L6 (260.2, 22.4305) -> (273.2, 22.4305)
  arc A7 (273.7, 21.9305) -> (273.2, 22.4305) centre (273.2, 21.9305) ccw
  line L7 (273.7, 21.9305) -> (273.7, 8.9305)
  arc A8 (202.55, 3.025) -> (203.05, 2.525) centre (203.05, 3.025) ccw
  line L8 (202.55, 3.025) -> (202.55, 16.025)
  arc A9 (203.05, 16.525) -> (202.55, 16.025) centre (203.05, 16.025) ccw
  line L9 (203.05, 16.525) -> (216.05, 16.525)
  arc A10 (216.55, 16.025) -> (216.05, 16.525) centre (216.05, 16.025) ccw
  line L10 (216.55, 16.025) -> (216.55, 3.025)
  arc A11 (216.05, 2.525) -> (216.55, 3.025) centre (216.05, 3.025) ccw
  line L11 (216.05, 2.525) -> (203.05, 2.525)
  arc A12 (177.95, 6.335) -> (178.45, 6.835) centre (177.95, 6.835) ccw
  line L12 (177.95, 6.335) -> (164.95, 6.335)
  arc A13 (164.45, 6.835) -> (164.95, 6.335) centre (164.95, 6.835) ccw
  line L13 (164.45, 6.835) -> (164.45, 19.835)
  arc A14 (164.95, 20.335) -> (164.45, 19.835) centre (164.95, 19.835) ccw
  line L14 (164.95, 20.335) -> (177.95, 20.335)
  arc A15 (178.45, 19.835) -> (177.95, 20.335) centre (177.95, 19.835) ccw
  line L15 (178.45, 19.835) -> (178.45, 6.835)
  arc A16 (221.6, 4.168) -> (222.1, 3.668) centre (222.1, 4.168) ccw
  line L16 (221.6, 4.168) -> (221.6, 17.168)
  arc A17 (222.1, 17.668) -> (221.6, 17.168) centre (222.1, 17.168) ccw
  line L17 (222.1, 17.668) -> (235.1, 17.668)
  arc A18 (235.6, 17.168) -> (235.1, 17.668) centre (235.1, 17.168) ccw
  line L18 (235.6, 17.168) -> (235.6, 4.168)
  arc A19 (235.1, 3.668) -> (235.6, 4.168) centre (235.1, 4.168) ccw
  line L19 (235.1, 3.668) -> (222.1, 3.668)
  arc A20 (240.65, 7.7875) -> (241.15, 7.2875) centre (241.15, 7.7875) ccw
  line L20 (240.65, 7.7875) -> (240.65, 20.7875)
  arc A21 (241.15, 21.2875) -> (240.65, 20.7875) centre (241.15, 20.7875) ccw
  line L21 (241.15, 21.2875) -> (254.15, 21.2875)
  arc A22 (254.65, 20.7875) -> (254.15, 21.2875) centre (254.15, 20.7875) ccw
  line L22 (254.65, 20.7875) -> (254.65, 7.7875)
  arc A23 (254.15, 7.2875) -> (254.65, 7.7875) centre (254.15, 7.7875) ccw
  line L23 (254.15, 7.2875) -> (241.15, 7.2875)
  line L24 (145.4, 54.46) -> (145.4, 67.46)
  arc A24 (145.9, 67.96) -> (145.4, 67.46) centre (145.9, 67.46) ccw
  line L25 (145.9, 67.96) -> (158.9, 67.96)
  arc A25 (159.4, 67.46) -> (158.9, 67.96) centre (158.9, 67.46) ccw
  line L26 (159.4, 67.46) -> (159.4, 54.46)
  arc A26 (158.9, 53.96) -> (159.4, 54.46) centre (158.9, 54.46) ccw
  line L27 (158.9, 53.96) -> (145.9, 53.96)
  arc A27 (145.4, 54.46) -> (145.9, 53.96) centre (145.9, 54.46) ccw
  arc A28 (183.5, 61.318) -> (184, 60.818) centre (184, 61.318) ccw
  line L28 (183.5, 61.318) -> (183.5, 74.318)
  arc A29 (184, 74.818) -> (183.5, 74.318) centre (184, 74.318) ccw
  line L29 (184, 74.818) -> (197, 74.818)
  arc A30 (197.5, 74.318) -> (197, 74.818) centre (197, 74.318) ccw
  line L30 (197.5, 74.318) -> (197.5, 61.318)
  arc A31 (197, 60.818) -> (197.5, 61.318) centre (197, 61.318) ccw
  line L31 (197, 60.818) -> (184, 60.818)
  line L32 (183.5, 23.218) -> (183.5, 36.218)
  arc A32 (184, 36.718) -> (183.5, 36.218) centre (184, 36.218) ccw
  line L33 (184, 36.718) -> (197, 36.718)
  arc A33 (197.5, 36.218) -> (197, 36.718) centre (197, 36.218) ccw
  line L34 (197.5, 36.218) -> (197.5, 23.218)
  arc A34 (197, 22.718) -> (197.5, 23.218) centre (197, 23.218) ccw
  line L35 (197, 22.718) -> (184, 22.718)
  arc A35 (183.5, 23.218) -> (184, 22.718) centre (184, 23.218) ccw
  arc A36 (164.45, 25.885) -> (164.95, 25.385) centre (164.95, 25.885) ccw
  line L36 (164.45, 25.885) -> (164.45, 38.885)
  arc A37 (164.95, 39.385) -> (164.45, 38.885) centre (164.95, 38.885) ccw
  line L37 (164.95, 39.385) -> (177.95, 39.385)
  arc A38 (178.45, 38.885) -> (177.95, 39.385) centre (177.95, 38.885) ccw
  line L38 (178.45, 38.885) -> (178.45, 25.885)
  arc A39 (177.95, 25.385) -> (178.45, 25.885) centre (177.95, 25.885) ccw
  line L39 (177.95, 25.385) -> (164.95, 25.385)
  arc A40 (202.55, 22.075) -> (203.05, 21.575) centre (203.05, 22.075) ccw
  line L40 (202.55, 22.075) -> (202.55, 35.075)
  arc A41 (203.05, 35.575) -> (202.55, 35.075) centre (203.05, 35.075) ccw
  line L41 (203.05, 35.575) -> (216.05, 35.575)
  arc A42 (216.55, 35.075) -> (216.05, 35.575) centre (216.05, 35.075) ccw
  line L42 (216.55, 35.075) -> (216.55, 22.075)
  arc A43 (216.05, 21.575) -> (216.55, 22.075) centre (216.05, 22.075) ccw
  line L43 (216.05, 21.575) -> (203.05, 21.575)
  arc A44 (240.65, 26.8375) -> (241.15, 26.3375) centre (241.15, 26.8375) ccw
  line L44 (240.65, 26.8375) -> (240.65, 39.8375)
  arc A45 (241.15, 40.3375) -> (240.65, 39.8375) centre (241.15, 39.8375) ccw
  line L45 (241.15, 40.3375) -> (254.15, 40.3375)
  arc A46 (254.65, 39.8375) -> (254.15, 40.3375) centre (254.15, 39.8375) ccw
  line L46 (254.65, 39.8375) -> (254.65, 26.8375)
  arc A47 (254.15, 26.3375) -> (254.65, 26.8375) centre (254.15, 26.8375) ccw
  line L47 (254.15, 26.3375) -> (241.15, 26.3375)
  arc A48 (221.6, 23.218) -> (222.1, 22.718) centre (222.1, 23.218) ccw
  line L48 (221.6, 23.218) -> (221.6, 36.218)
  arc A49 (222.1, 36.718) -> (221.6, 36.218) centre (222.1, 36.218) ccw
  line L49 (222.1, 36.718) -> (235.1, 36.718)
  arc A50 (235.6, 36.218) -> (235.1, 36.718) centre (235.1, 36.218) ccw
  line L50 (235.6, 36.218) -> (235.6, 23.218)
  arc A51 (235.1, 22.718) -> (235.6, 23.218) centre (235.1, 23.218) ccw
  line L51 (235.1, 22.718) -> (222.1, 22.718)
  arc A52 (202.55, 41.125) -> (203.05, 40.625) centre (203.05, 41.125) ccw
  line L52 (202.55, 41.125) -> (202.55, 54.125)
  arc A53 (203.05, 54.625) -> (202.55, 54.125) centre (203.05, 54.125) ccw
  line L53 (203.05, 54.625) -> (216.05, 54.625)
  arc A54 (216.55, 54.125) -> (216.05, 54.625) centre (216.05, 54.125) ccw
  line L54 (216.55, 54.125) -> (216.55, 41.125)
  arc A55 (216.05, 40.625) -> (216.55, 41.125) centre (216.05, 41.125) ccw
  line L55 (216.05, 40.625) -> (203.05, 40.625)
  arc A56 (221.6, 42.268) -> (222.1, 41.768) centre (222.1, 42.268) ccw
  line L56 (221.6, 42.268) -> (221.6, 55.268)
  arc A57 (222.1, 55.768) -> (221.6, 55.268) centre (222.1, 55.268) ccw
  line L57 (222.1, 55.768) -> (235.1, 55.768)
  arc A58 (235.6, 55.268) -> (235.1, 55.768) centre (235.1, 55.268) ccw
  line L58 (235.6, 55.268) -> (235.6, 42.268)
  arc A59 (235.1, 41.768) -> (235.6, 42.268) centre (235.1, 42.268) ccw
  line L59 (235.1, 41.768) -> (222.1, 41.768)
  line L60 (259.7, 27.9805) -> (259.7, 40.9805)
  arc A60 (260.2, 41.4805) -> (259.7, 40.9805) centre (260.2, 40.9805) ccw
  line L61 (260.2, 41.4805) -> (273.2, 41.4805)
  arc A61 (273.7, 40.9805) -> (273.2, 41.4805) centre (273.2, 40.9805) ccw
  line L62 (273.7, 40.9805) -> (273.7, 27.9805)
  arc A62 (273.2, 27.4805) -> (273.7, 27.9805) centre (273.2, 27.9805) ccw
  line L63 (273.2, 27.4805) -> (260.2, 27.4805)
  arc A63 (259.7, 27.9805) -> (260.2, 27.4805) centre (260.2, 27.9805) ccw
  arc A64 (183.5, 42.268) -> (184, 41.768) centre (184, 42.268) ccw
  line L64 (183.5, 42.268) -> (183.5, 55.268)
  arc A65 (184, 55.768) -> (183.5, 55.268) centre (184, 55.268) ccw
  line L65 (184, 55.768) -> (197, 55.768)
  arc A66 (197.5, 55.268) -> (197, 55.768) centre (197, 55.268) ccw
  line L66 (197.5, 55.268) -> (197.5, 42.268)
  arc A67 (197, 41.768) -> (197.5, 42.268) centre (197, 42.268) ccw
  line L67 (197, 41.768) -> (184, 41.768)
  arc A68 (240.65, 45.8875) -> (241.15, 45.3875) centre (241.15, 45.8875) ccw
  line L68 (240.65, 45.8875) -> (240.65, 58.8875)
  arc A69 (241.15, 59.3875) -> (240.65, 58.8875) centre (241.15, 58.8875) ccw
  line L69 (241.15, 59.3875) -> (254.15, 59.3875)
  arc A70 (254.65, 58.8875) -> (254.15, 59.3875) centre (254.15, 58.8875) ccw
  line L70 (254.65, 58.8875) -> (254.65, 45.8875)
  arc A71 (254.15, 45.3875) -> (254.65, 45.8875) centre (254.15, 45.8875) ccw
  line L71 (254.15, 45.3875) -> (241.15, 45.3875)
  arc A72 (177.95, 44.435) -> (178.45, 44.935) centre (177.95, 44.935) ccw
  line L72 (177.95, 44.435) -> (164.95, 44.435)
  arc A73 (164.45, 44.935) -> (164.95, 44.435) centre (164.95, 44.935) ccw
  line L73 (164.45, 44.935) -> (164.45, 57.935)
  arc A74 (164.95, 58.435) -> (164.45, 57.935) centre (164.95, 57.935) ccw
  line L74 (164.95, 58.435) -> (177.95, 58.435)
  arc A75 (178.45, 57.935) -> (177.95, 58.435) centre (177.95, 57.935) ccw
  line L75 (178.45, 57.935) -> (178.45, 44.935)
  arc A76 (193.025, 81.7015) -> (193.525, 81.2015) centre (193.525, 81.7015) ccw
  line L76 (193.025, 81.7015) -> (193.025, 94.7015)
  arc A77 (193.525, 95.2015) -> (193.025, 94.7015) centre (193.525, 94.7015) ccw
  line L77 (193.525, 95.2015) -> (206.525, 95.2015)
  arc A78 (207.025, 94.7015) -> (206.525, 95.2015) centre (206.525, 94.7015) ccw
  line L78 (207.025, 94.7015) -> (207.025, 81.7015)
  arc A79 (206.525, 81.2015) -> (207.025, 81.7015) centre (206.525, 81.7015) ccw
  line L79 (206.525, 81.2015) -> (193.525, 81.2015)
  arc A80 (225.575, 81.2015) -> (226.075, 81.7015) centre (225.575, 81.7015) ccw
  line L80 (225.575, 81.2015) -> (212.575, 81.2015)
  arc A81 (212.075, 81.7015) -> (212.575, 81.2015) centre (212.575, 81.7015) ccw
  line L81 (212.075, 81.7015) -> (212.075, 94.7015)
  arc A82 (212.575, 95.2015) -> (212.075, 94.7015) centre (212.575, 94.7015) ccw
  line L82 (212.575, 95.2015) -> (225.575, 95.2015)
  arc A83 (226.075, 94.7015) -> (225.575, 95.2015) centre (225.575, 94.7015) ccw
  line L83 (226.075, 94.7015) -> (226.075, 81.7015)
  arc A84 (221.6, 61.318) -> (222.1, 60.818) centre (222.1, 61.318) ccw
  line L84 (221.6, 61.318) -> (221.6, 74.318)
  arc A85 (222.1, 74.818) -> (221.6, 74.318) centre (222.1, 74.318) ccw
  line L85 (222.1, 74.818) -> (235.1, 74.818)
  arc A86 (235.6, 74.318) -> (235.1, 74.818) centre (235.1, 74.318) ccw
  line L86 (235.6, 74.318) -> (235.6, 61.318)
  arc A87 (235.1, 60.818) -> (235.6, 61.318) centre (235.1, 61.318) ccw
  line L87 (235.1, 60.818) -> (222.1, 60.818)
  arc A88 (164.45, 63.985) -> (164.95, 63.485) centre (164.95, 63.985) ccw
  line L88 (164.45, 63.985) -> (164.45, 76.985)
  arc A89 (164.95, 77.485) -> (164.45, 76.985) centre (164.95, 76.985) ccw
  line L89 (164.95, 77.485) -> (177.95, 77.485)
  arc A90 (178.45, 76.985) -> (177.95, 77.485) centre (177.95, 76.985) ccw
  line L90 (178.45, 76.985) -> (178.45, 63.985)
  arc A91 (177.95, 63.485) -> (178.45, 63.985) centre (177.95, 63.985) ccw
  line L91 (177.95, 63.485) -> (164.95, 63.485)
  arc A92 (240.65, 64.9375) -> (241.15, 64.4375) centre (241.15, 64.9375) ccw
  line L92 (240.65, 64.9375) -> (240.65, 77.9375)
  arc A93 (241.15, 78.4375) -> (240.65, 77.9375) centre (241.15, 77.9375) ccw
  line L93 (241.15, 78.4375) -> (254.15, 78.4375)
  arc A94 (254.65, 77.9375) -> (254.15, 78.4375) centre (254.15, 77.9375) ccw
  line L94 (254.65, 77.9375) -> (254.65, 64.9375)
  arc A95 (254.15, 64.4375) -> (254.65, 64.9375) centre (254.15, 64.9375) ccw
  line L95 (254.15, 64.4375) -> (241.15, 64.4375)
  arc A96 (259.7, 47.0305) -> (260.2, 46.5305) centre (260.2, 47.0305) ccw
  line L96 (259.7, 47.0305) -> (259.7, 60.0305)
  arc A97 (260.2, 60.5305) -> (259.7, 60.0305) centre (260.2, 60.0305) ccw
  line L97 (260.2, 60.5305) -> (273.2, 60.5305)
  arc A98 (273.7, 60.0305) -> (273.2, 60.5305) centre (273.2, 60.0305) ccw
  line L98 (273.7, 60.0305) -> (273.7, 47.0305)
  arc A99 (273.2, 46.5305) -> (273.7, 47.0305) centre (273.2, 47.0305) ccw
  line L99 (273.2, 46.5305) -> (260.2, 46.5305)
  arc A100 (202.55, 60.175) -> (203.05, 59.675) centre (203.05, 60.175) ccw
  line L100 (202.55, 60.175) -> (202.55, 73.175)
  arc A101 (203.05, 73.675) -> (202.55, 73.175) centre (203.05, 73.175) ccw
  line L101 (203.05, 73.675) -> (216.05, 73.675)
  arc A102 (216.55, 73.175) -> (216.05, 73.675) centre (216.05, 73.175) ccw
  line L102 (216.55, 73.175) -> (216.55, 60.175)
  arc A103 (216.05, 59.675) -> (216.55, 60.175) centre (216.05, 60.175) ccw
  line L103 (216.05, 59.675) -> (203.05, 59.675)
  arc A104 (173.975, 83.035) -> (174.475, 82.535) centre (174.475, 83.035) ccw
  line L104 (173.975, 83.035) -> (173.975, 96.035)
  arc A105 (174.475, 96.535) -> (173.975, 96.035) centre (174.475, 96.035) ccw
  line L105 (174.475, 96.535) -> (187.475, 96.535)
  arc A106 (187.975, 96.035) -> (187.475, 96.535) centre (187.475, 96.035) ccw
  line L106 (187.975, 96.035) -> (187.975, 83.035)
  arc A107 (187.475, 82.535) -> (187.975, 83.035) centre (187.475, 83.035) ccw
  line L107 (187.475, 82.535) -> (174.475, 82.535)
  arc A108 (259.7, 66.0805) -> (260.2, 65.5805) centre (260.2, 66.0805) ccw
  line L108 (259.7, 66.0805) -> (259.7, 79.0805)
  arc A109 (260.2, 79.5805) -> (259.7, 79.0805) centre (260.2, 79.0805) ccw
  line L109 (260.2, 79.5805) -> (273.2, 79.5805)
  arc A110 (273.7, 79.0805) -> (273.2, 79.5805) centre (273.2, 79.0805) ccw
  line L110 (273.7, 79.0805) -> (273.7, 66.0805)
  arc A111 (273.2, 65.5805) -> (273.7, 66.0805) centre (273.2, 66.0805) ccw
  line L111 (273.2, 65.5805) -> (260.2, 65.5805)
  line L112 (151.218, 98.3323) -> (164.0701, 92.7802)
  line L113 (164.0701, 92.7802) -> (158.518, 79.9282)
  line L114 (158.518, 79.9282) -> (145.666, 85.4803)
  line L115 (145.666, 85.4803) -> (151.218, 98.3323)
  arc A112 (226.8375, 1.725) -> (274.5, 6.8214) centre (226.8375, 227.1492) ccw
  line L116 (274.5, 6.8214) -> (274.5, 80.3805)
  line L117 (274.5, 80.3805) -> (226.875, 80.3805)
  line L118 (226.875, 80.3805) -> (226.875, 97.335)
  line L119 (226.875, 97.335) -> (165.6302, 97.335)
  line L120 (165.6302, 97.335) -> (152.3872, 103.056)
  line L121 (152.3872, 103.056) -> (145.4689, 87.0414)
  arc A113 (145.4689, 87.0414) -> (140.8942, 64.9159) centre (196.6857, 64.9159) ccw
  line L122 (140.8942, 64.9159) -> (140.8942, 1.725)
  line L123 (140.8942, 1.725) -> (226.8375, 1.725)
  line L124 (178.45, 7.2444) -> (183.5, 7.2444)
  line L125 (254.65, 9.189) -> (259.7, 9.189)
  line L126 (269.2916, 65.5805) -> (269.2916, 60.5305)
  line L127 (207.025, 92.3887) -> (212.075, 92.3887)
  line L128 (141.8525, 75.2122) -> (145.8174, 74.0025)
  line L129 (145.8174, 74.0025) -> (147.0597, 78.0742)
  line L130 (147.0597, 78.0742) -> (142.8001, 79.3739)
  line L131 (207.025, 92.3887) -> (207.025, 97.335)
  line L132 (212.075, 92.3887) -> (212.075, 97.335)
  line L133 (269.2916, 65.5805) -> (274.5, 65.5805)
  line L134 (269.2916, 60.5305) -> (274.5, 60.5305)
  line L135 (254.65, 9.189) -> (254.65, 3.4473)
  line L136 (259.7, 9.189) -> (259.7, 4.1332)
  line L137 (178.45, 7.2444) -> (178.45, 1.725)
  line L138 (183.5, 7.2444) -> (183.5, 1.725)
  constraint coincident L15 L124.start
  constraint coincident L0 L124.end
  constraint perpendicular L0 L124
  constraint coincident L22 L125.start
  constraint coincident L5 L125.end
  constraint perpendicular L5 L125
  constraint coincident L111 L126.start
  constraint coincident L97 L126.end
  constraint perpendicular L97 L126
  constraint coincident L78 L127.start
  constraint coincident L81 L127.end
  constraint perpendicular L81 L127
  constraint coincident A113 L128.start
  constraint perpendicular L128 L129
  constraint coincident A113 L130.end
  constraint perpendicular L129 L130
  constraint coincident L119 L131.end
  constraint perpendicular L119 L131
  constraint coincident L119 L132.end
  constraint perpendicular L119 L132
  constraint coincident L116 L133.end
  constraint perpendicular L116 L133
  constraint coincident L116 L134.end
  constraint perpendicular L116 L134
  constraint coincident A112 L135.end
  constraint perpendicular L134 L135
  constraint coincident A112 L136.end
  constraint perpendicular L125 L136
  constraint coincident L123 L137.end
  constraint perpendicular L123 L137
  constraint coincident L123 L138.end
  constraint perpendicular L123 L138
extrude "Extrude5" add sketch "Sketch6" along normal blind 11 contours L0 L15 L123 L124 L137 L138 | L5 L22 A112 L125 L135 L136 | A113 L128 L129 L130 | L97 L111 L116 L126 L133 L134 | L78 L81 L119 L127 L131 L132 bodies 1